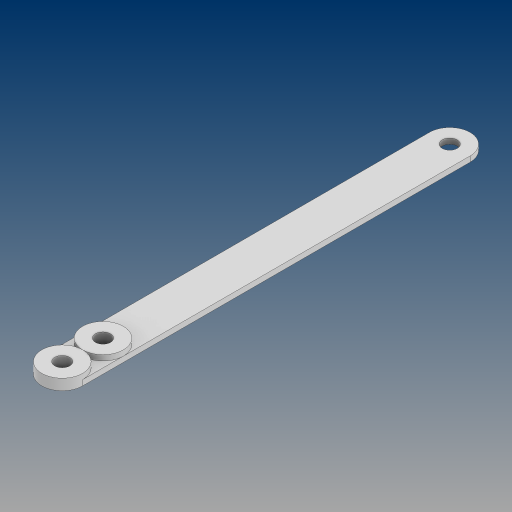
# Autodesk Inventor part: közeplsoszalag1
Saved by Autodesk Inventor 2023 (Build 270158000, 158)
## iProperties
Created: 2023-11-15
Part Number: közeplsoszalag1
Material: Generic
Document SubType Name: Modeling
Designer: gd1
Density: 1 g/cm^3
Appearance: Default
Author: gd1
Autodesk Inventor part; units mm, degrees
ref_plane "YZ Plane" through (0, 0, 0) normal (1, 0, 0) x (0, 1, 0)
ref_plane "XZ Plane" through (0, 0, 0) normal (0, 1, 0) x (-1, 0, 0)
ref_plane "XY Plane" through (0, 0, 0) normal (0, 0, 1) x (1, 0, 0)
sketch "Sketch1" plane through (0, 0, 0) normal (0, 1, 0) x (-1, 0, 0)
  line L0 (0, 0) -> (15, 0)
  line L1 (15, 0) -> (15, -30)
  line L2 (15, -30) -> (0, -30)
  line L3 (0, -30) -> (0, 0)
  line L4 (7.5, 0) -> (7.5, -157.6812)
  line L5 (7.5, 0) -> (165.1812, 0) construction
  line L6 (7.5, -157.6812) -> (7.5, -150.1812)
  circle A0 centre (7.5, -150.1812) radius 7.5
  circle A1 centre (7.5, -7.5) radius 7.5
  circle A2 centre (7.5, -22.5) radius 7.5
  circle A3 centre (7.5, -7.5) radius 2.75
  line L7 (15, 0) -> (0, 0)
  line L8 (0, 0) -> (0, -157.6812)
  line L9 (0, -157.6812) -> (15, -157.6812)
  line L10 (15, -157.6812) -> (15, 0)
  circle A4 centre (7.5, -150.1812) radius 2.75
  circle A5 centre (7.5, -22.5) radius 2.75
  point P0 (0, -150.1812)
  point P1 (15, -150.1812)
  point P2 (15, -7.5)
  point P3 (0, -7.5)
  point P4 (7.5, -15)
  dimension "d9" = 15
  dimension "d10" = 30
  dimension "d11" = 157.6812
  dimension "d12" = 90
  dimension "d13" = 7.5
  dimension "d14" = 15
  dimension "d15" = 15
  dimension "d16" = 15
  dimension "d17" = 5.5
  dimension "d18" = 5.5
  dimension "d19" = 5.5
  constraints: 22 end point, 6 centre point, 4 coincident, 4 parallel, 4 tangent, 3 horizontal, 3 perpendicular, 1 midpoint, 1 point on line, 1 vertical
  measures "d9" distance of L1.end L2.end
  measures "d10" distance of L0.end L1.end
  measures "d11" distance of L4.start L4.end
  measures "d12" angle of L4 L5
  measures "d13" distance of L4.end L6.end
  measures "d14" diameter of A0
  measures "d15" diameter of A1
  measures "d16" diameter of A2
  measures "d17" diameter of A3
  measures "d18" diameter of A4
  measures "d19" diameter of A5
extrude "Extrusion1" add sketch "Sketch1" along normal blind 2 contours A1 L4 A3 | L4 A3 A1 | A1 A2 L3 | L1 A2 A1 | A2 L2 L3 | A2 L4 A5 | A2 L4 A5 | L1 L2 A2 | L2 L4 A0 L8 | L2 L10 A0 L4 | A0 L4 A4 | A0 L4 A4
extrude "Extrusion2" add sketch "Sketch1" along normal blind 3 contours A1 L4 A3 | L4 A3 A1 | A2 L4 A5 | A2 L4 A5
extrude "Extrusion3" cut sketch "Sketch1" along normal mid plane 2 contours A3 L4 | L4 A3 | A5 L4 | L4 A5 | A4 L4 | L4 A4
extrude "Extrusion4" add sketch "Sketch1" along normal blind 4 contours A1 L4 A3 | L4 A3 A1 | A2 L4 A5 | A2 L4 A5
body "Solid1"
